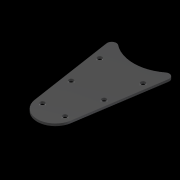
# Autodesk Inventor part: JointD0cover_2nd
Saved by Autodesk Inventor 2011 (Build 150239000, 239)
## iProperties
Created: 2013-02-08
Part Number: JointD0cover_2nd
Document SubType Name: Modeling
Designer: JohnHenry
Density: 1 g/cm^3
Author: JohnHenry
Autodesk Inventor part; units mm, degrees
ref_plane "YZ Plane" through (0, 0, 0) normal (1, 0, 0) x (0, 1, 0)
ref_plane "XZ Plane" through (0, 0, 0) normal (0, 1, 0) x (-1, 0, 0)
ref_plane "XY Plane" through (0, 0, 0) normal (0, 0, 1) x (1, 0, 0)
sketch "スケッチ1" plane through (0, 0, 0) normal (0, 0, 1) x (1, 0, 0)
  circle A0 centre (4.9426, -52.053) radius 1
  circle A1 centre (7.2088, -37.2252) radius 1
  circle A2 centre (9.475, -22.3974) radius 1
  circle A3 centre (-7.2088, -37.2252) radius 1
  circle A4 centre (-4.9426, -52.053) radius 1
  circle A5 centre (-9.475, -22.3974) radius 1
  arc A6 (13.5882, -15.3415) -> (10.3889, -13.4562) centre (11.6111, -15.0393) ccw
  arc A7 (-10.3889, -13.4562) -> (10.3889, -13.4562) centre (0, 0) ccw
  arc A8 (-10.3889, -13.4562) -> (-13.5882, -15.3415) centre (-11.6111, -15.0393) ccw
  line L0 (-7.9082, -52.5063) -> (-13.5882, -15.3415)
  arc A9 (-7.9082, -52.5063) -> (-1.1, -59.2216) centre (0, -51.2976) ccw
  arc A10 (1.1, -59.2216) -> (7.9082, -52.5063) centre (0, -51.2976) ccw
  line L1 (13.5882, -15.3415) -> (7.9082, -52.5063)
  arc A11 (-7.9082, -52.5063) -> (7.9082, -52.5063) centre (0, -51.2976) ccw
  constraints: 12 centre point, 12 point on circle, 4 end point, 1 coincident, 1 concentric
extrude "押し出し1" add sketch "スケッチ1" along normal blind 1
